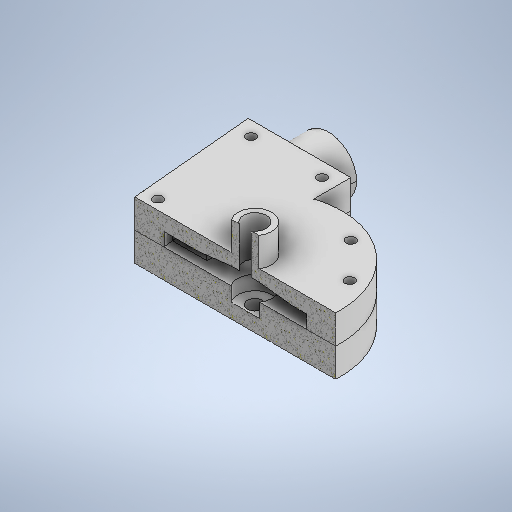
# Autodesk Inventor part: Voluta
Saved by Autodesk Inventor 2025.3 (Build 293356000, 356)
## iProperties
Created: 2025-11-12
Part Number: Voluta
Material: Generic
Document SubType Name: Modeling
Designer: juanm
Density: 1 g/cm^3
Appearance: Default
Author: juanm
Autodesk Inventor part; units mm, degrees
ref_plane "YZ Plane" through (0, 0, 0) normal (1, 0, 0) x (0, 1, 0)
ref_plane "XZ Plane" through (0, 0, 0) normal (0, 1, 0) x (-1, 0, 0)
ref_plane "XY Plane" through (0, 0, 0) normal (0, 0, 1) x (1, 0, 0)
sketch "Sketch1" plane through (0, 0, 0) normal (0, 1, 0) x (-1, 0, 0)
  circle A0 centre (0, 0) radius 25
  line L0 (0, 0) -> (25, 0) construction
  line L1 (0, 0) -> (19.1511, 16.0697) construction
  line L2 (0, 0) -> (4.3412, 24.6202) construction
  line L3 (0, 0) -> (-12.5, 21.6506) construction
  line L4 (0, 0) -> (-23.4923, 8.5505) construction
  line L5 (0, 0) -> (-23.4923, -8.5505) construction
  line L6 (0, 0) -> (-12.5, -21.6506) construction
  line L7 (0, 0) -> (4.3412, -24.6202) construction
  line L8 (0, 0) -> (19.1511, -16.0697) construction
  line L9 (19.1511, -16.0697) -> (19.4575, -16.3268)
  line L10 (4.3412, -24.6202) -> (4.7059, -26.6883)
  line L11 (-12.5, -21.6506) -> (-14.5, -25.1147)
  line L12 (-23.4923, -8.5505) -> (-29.1305, -10.6026)
  line L13 (-23.4923, 8.5505) -> (-31.0099, 11.2867)
  line L14 (-12.5, 21.6506) -> (-17.5, 30.3109)
  line L15 (4.3412, 24.6202) -> (6.425, 36.4379)
  line L16 (19.1511, 16.0697) -> (30.6418, 25.7115)
  line L17 (25, 0) -> (43, 0) construction
  spline S0 degree 4 poles (25, 0) (24.7233, -10.5773) (16.303, -28.2482) (-10.9374, -33.3792) (-32.4895, -11.3227) (-34.2694, 12.9576) (-12.7094, 42.562) (23.8605, 39.8981) (41.7423, 18.3571) (43, 0) knots 0 0 0 0 0 0.252149 0.357713 0.466731 0.579176 0.695209 1 1 1 1 1
  line L18 (43, 0) -> (58, 0)
  line L19 (30.6418, 25.7115) -> (42.1324, 35.3533)
  line L20 (6.425, 36.4379) -> (9.0297, 51.21)
  line L21 (-17.5, 30.3109) -> (-25, 43.3013)
  line L22 (-31.0099, 11.2867) -> (-45.1052, 16.417)
  line L23 (-29.1305, -10.6026) -> (-43.2259, -15.7329)
  line L24 (-14.5, -25.1147) -> (-22, -38.1051)
  line L25 (4.7059, -26.6883) -> (7.3106, -41.4604)
  line L26 (19.4575, -16.3268) -> (30.9482, -25.9686)
  spline S1 degree 4 poles (30.9482, -25.9686) (20.5729, -40.5703) (-9.4837, -52.4783) (-47.5087, -29.6861) (-49.8324, 18.6263) (-18.2766, 60.1903) (33.0838, 55.9088) (56.8657, 24.7753) (58, 0) knots 0 0 0 0 0 0.295562 0.417688 0.542421 0.669901 1 1 1 1 1
  line L27 (48.5, -60) -> (25, -60)
  line L28 (25, 0) -> (25, -60)
  line L29 (48.5, -60) -> (43, 0)
  line L30 (48.5, -60) -> (63.5, -60)
  line L31 (63.5, -60) -> (58, 0)
  line L32 (25, -60) -> (10, -60)
  line L33 (10, -60) -> (10, -40.7262)
  line L34 (43, 0) -> (25, 0)
  point P0 (25.3488, -21.2701)
  point P1 (6.0082, -34.0743)
  point P2 (-18.25, -31.6099)
  point P3 (-36.1782, -13.1678)
  point P4 (-38.0576, 13.8518)
  point P5 (-21.25, 36.8061)
  point P6 (7.7273, 43.8239)
  point P7 (36.3871, 30.5324)
  point P8 (50.5, 0)
  point P9 (22.9315, -9.9573)
  dimension "d0" = 50
  dimension "d3" = 360
  dimension "d5" = 25.4
  dimension "d6" = 27.1
  dimension "d7" = 29
  dimension "d8" = 33
  dimension "d9" = 35
  dimension "d10" = 37
  dimension "d11" = 40
  dimension "d12" = 43
  dimension "d13" = 31
  dimension "d14" = 15
  dimension "d15" = 15
  dimension "d16" = 15
  dimension "d17" = 15
  dimension "d18" = 15
  dimension "d19" = 15
  dimension "d20" = 15
  dimension "d21" = 15
  dimension "d22" = 15
  dimension "d23" = 23.5
  dimension "d24" = 60
  dimension "d25" = 15
  dimension "d26" = 15
  constraints: 70 end point, 16 collinear, 8 midpoint, 6 horizontal, 2 point on line, 2 vertical, 1 coincident, 1 perpendicular, 52 other
  measures "d5" distance of L9.end point (0, 0)
  measures "d6" distance of L10.end point (0, 0)
  measures "d7" distance of point (0, 0) L11.end
  measures "d8" distance of point (0, 0) L13.end
  measures "d9" distance of L3.start L14.end
  measures "d10" distance of point (0, 0) L15.end
  measures "d11" distance of L16.end L2.start
  measures "d12" distance of L5.start L17.end
  measures "d13" distance of point (0, 0) L12.end
  measures "d14" distance of L17.end L18.end
  measures "d15" distance of L16.end L19.end
  measures "d16" distance of L15.end L20.end
  measures "d17" distance of L14.end L21.end
  measures "d18" distance of L13.end L22.end
  measures "d19" distance of L12.end L23.end
  measures "d20" distance of L11.end L24.end
  measures "d21" distance of L10.end L25.end
  measures "d22" distance of L9.end L26.end
  measures "d23" distance of L27.start L27.end
  measures "d24" distance of L0.end L27.end
  measures "d25" distance of L27.start L30.end
  measures "d26" distance of L27.end L32.end
extrude "Extrusion1" add sketch "Sketch1" against normal blind 15
extrude "Extrusion2" add sketch "Sketch1" along normal blind 7 contours L28 L26 S0 A0 | L34 L29 L27 L28 S1 L26 | L28 S1 L25 S0 L26 | L26 S1 L28 | S0 L19 S1 L18 | L18 L31 L30 L29 | S0 L20 S1 L19 | L28 L32 L33 S1 | S0 L21 S1 L20 | L25 S1 L24 S0 | S0 L22 S1 L21 | L24 S1 L23 S0 | S0 L23 S1 L22
sketch "Sketch2" plane through (0, 7, 0) normal (0, 1, 0) x (1, 0, 0)
  line L0 (-10, 40.7262) -> (-10, 60) projected
  arc A0 (-22.9315, 9.9573) -> (-25, 0) centre (0, 0) ccw projected
  line L1 (-63.5, 60) -> (-58, 0) projected
  spline S0 degree 4 poles (-58, 0) (-56.8657, -24.7753) (-33.0838, -55.9088) (18.2766, -60.1903) (49.8324, -18.6263) (47.8717, 22.1387) (22.8112, 43.0756) (1.5485, 44.2841) (-10, 40.7262) knots 0 0 0 0 0 0.368682 0.511063 0.650376 0.786777 1 1 1 1 1 projected
  arc A1 (-22.9315, 9.9573) -> (-25, 0) centre (0, 0) ccw projected
  line L2 (-25, 0) -> (-43, 0)
  line L3 (-25, 0) -> (-43, 0) projected
  line L4 (-10, 60) -> (-63.5, 60) projected
  line L5 (-43, 0) -> (-25, 0) projected
  constraints: 2 end point, 1 horizontal, 3 other
extrude "Extrusion3" add sketch "Sketch2" along normal blind 8
sketch "Sketch4" plane through (-10, -15, -60) normal (0, 0, -1) x (-1, 0, 0)
  line L0 (38.5, 15) -> (15, 15) projected
  circle A0 centre (26.75, 15) radius 11.75
  circle A1 centre (26.75, 15) radius 14.75
  point P0 (-10, 15)
  dimension "d33" = 3
  constraints: 1 centre point, 1 coincident, 1 horizontal alignment, 1 midpoint, 2 other
extrude "Extrusion4" add sketch "Sketch4" along normal blind 15
loft "Loft1" cut section 1 edges at (-34, 0, 0) (-25, 3.5, 0) (-34, 7, 0) (-43, 3.5, 0) section 2 edges at (-25, 0, -60)
sketch "Sketch5" plane through (0, -15, 0) normal (0, -1, 0) x (1, 0, 0)
  circle A0 centre (0, 0) radius 4
  dimension "d48" = 8
  constraints: 1 centre point, 1 coincident
  measures "d48" diameter of A0
extrude "Extrusion5" cut sketch "Sketch5" against normal blind 20
sketch "Sketch6" plane through (0, 0, 0) normal (0, 0, 1) x (1, 0, 0)
  line L0 (0, 0) -> (0, 10)
  line L1 (0, 0) -> (-25, 0)
  line L2 (-4, 0) -> (4, 0) projected
  line L3 (-25, 0) -> (-25, 7)
  line L4 (-25, 7) -> (0, 10)
  point P0 (-22.9315, 0)
  dimension "d51" = 10
  dimension "d52" = 25
  dimension "d54" = 7
  constraints: 8 end point, 1 collinear, 1 vertical
  measures "d51" distance of L0.start L0.end
  measures "d52" distance of L0.start L1.end
  measures "d54" distance of L1.end L3.end
revolve "Revolution1" cut sketch "Sketch6" angle 360 about axis through (0, 0, 0) along (0, 1, 0)
sketch "Sketch8" plane through (0, 15, 0) normal (0, 1, 0) x (1, 0, 0)
  circle A0 centre (0, 0) radius 8.75
  dimension "d58" = 17.5
  constraints: 1 centre point, 1 coincident
  measures "d58" diameter of A0
extrude "Extrusion7" cut sketch "Sketch8" against normal blind 10
sketch "Sketch9" plane through (0, 0, 0) normal (0, 1, 0) x (1, 0, 0)
  circle A0 centre (0, 0) radius 4 projected
  circle A1 centre (0, 0) radius 9
  dimension "d61" = 18
  constraints: 1 centre point, 1 coincident
  measures "d61" diameter of A1
extrude "Extrusion8" cut sketch "Sketch9" against normal blind 7.4
sketch "Sketch10" plane through (0, 15, 0) normal (0, 1, 0) x (1, 0, 0)
  line L0 (-10, 60) -> (-10, 40.7262) projected
  line L1 (-63.5, 60) -> (-58, 0) projected
  line L2 (-48.5, 60) -> (-63.5, 60) projected
  line L3 (-25, 60) -> (-10, 60) projected
  line L4 (-25, 0) -> (-25, 60) projected
  line L5 (-48.5, 60) -> (-43, 0) projected
  point P0 (0, 0)
  point P1 (-50.5, 0)
  point P2 (-36.3871, -30.5324)
  point P3 (-7.7273, -43.8239)
  point P4 (21.25, -36.8061)
  point P5 (38.0576, -13.8518)
  point P6 (36.1782, 13.1678)
  point P7 (18.25, 31.6099)
  point P8 (-6.0082, 34.0743)
  point P9 (-54.5, 52.5)
  point P10 (-17.5, 52.5)
  dimension "d64" = 7.5
  dimension "d65" = 7.5
  dimension "d66" = 7.5
  dimension "d67" = 6
  measures "d64" distance from line of L0 point (-17.5, 52.5)
  measures "d65" distance from line of L3 point (-17.5, 52.5)
  measures "d66" distance from line of L2 point (-54.5, 52.5)
  measures "d67" horizontal distance of L2.start point (-54.5, 52.5)
hole "Hole2" at (-17.5, 15, -52.5) at (-54.5, 15, -52.5) at (-50.5, 15, 0) at (-36.3871, 15, 30.5324) at (-7.7273, 15, 43.8239) at (21.25, 15, 36.8061) at (38.0576, 15, 13.8518) at (36.1782, 15, -13.1678) at (18.25, 15, -31.6099) direction (0, -1, 0) diameter 5 end through all
split body "Split1" result two bodies by plane through (0, 0, 0) normal (0, 1, 0) first body at (-40.4461, 14.5, -34.4904)
sketch "Sketch11" plane through (0, 15, 0) normal (0, 1, 0) x (1, 0, 0)
  circle A0 centre (0, 0) radius 8.75 projected
  circle A1 centre (0, 0) radius 5.95
  dimension "d87" = 2.8
  constraints: 1 centre point, 1 coincident
  measures "d87" radial gap between concentric circles of A0 A1
extrude "Extrusion9" add sketch "Sketch11" along normal blind 15 and the other way blind 6 bodies 2
body "Solid2"
body "Solid3"
